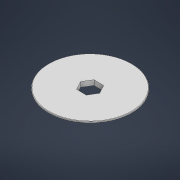
# Autodesk Inventor part: Pulley because david still hates it
Saved by Autodesk Inventor 2022 (Build 260153000, 153)
## iProperties
Created: 2022-01-21
Part Number: Pulley because david still hates it
Material: Generic
Document SubType Name: Modeling
Designer: izack
Density: 1 g/cm^3
Appearance: Default
Author: izack
## iProperties of the stored document Pulley because david hates it_3DPrint.ipt
Created: 2022-01-21
Part Number: Pulley because david hates it_3DPrint
Material: Generic
Document SubType Name: Modeling
Designer: izack
Density: 1 g/cm^3
Appearance: Default
Author: izack
Autodesk Inventor part; units mm, degrees
ref_plane "YZ Plane" through (0, 0, 0) normal (1, 0, 0) x (0, 1, 0)
ref_plane "XZ Plane" through (0, 0, 0) normal (0, 1, 0) x (-1, 0, 0)
ref_plane "XY Plane" through (0, 0, 0) normal (0, 0, 1) x (1, 0, 0)
sketch "Sketch1" plane through (0, 0, 0) normal (0, 0, 1) x (1, 0, 0)
  line L0 (0, 0) -> (12.7, 0)
  line L1 (12.7, 0) -> (12.7, 3)
  line L2 (12.7, 3) -> (0, 3)
  line L3 (0, 3) -> (0, 0)
  ellipse E0 centre (12.7, 1.5) end of major axis (9.9101, 1.5) minor radius 0.9957
  point P0 (12.7, 0.5043)
  point P1 (12.7, 2.4957)
  dimension "d0" = 12.7
  dimension "d1" = 3
  constraints: 8 end point, 3 perpendicular, 1 horizontal, 1 midpoint, 2 other
  measures "d0" distance of L0.start L0.end
  measures "d1" distance of L0.end L1.end
revolve "Revolution1" add sketch "Sketch1" angle 360 about axis through (0, 3, 0) along (0, -1, 0) contours L3 L2 L1 E0 L0
fillet "Fillet1" radius 0.127 4 edges at (-12.7, 3, 0) (-12.7, 2.4957, 0) (-12.7, 0.5043, 0) (-12.7, 0, 0)
sketch "Sketch2" plane through (0, 0, 0) normal (0, -1, 0) x (1, 0, 0)
  circle A0 centre (0, 0) radius 2.6
  line L0 (1.5658, -2.5616) -> (-1.4355, -2.6368)
  line L1 (-1.4355, -2.6368) -> (-3.0013, -0.0752)
  line L2 (-3.0013, -0.0752) -> (-1.5658, 2.5616)
  line L3 (-1.5658, 2.5616) -> (1.4355, 2.6368)
  line L4 (1.4355, 2.6368) -> (3.0013, 0.0752)
  line L5 (3.0013, 0.0752) -> (1.5658, -2.5616)
  point P0 (2.2835, -1.2432)
  dimension "d4" = 5.2
  constraints: 12 end point, 2 coincident, 1 midpoint, 16 other
extrude "Extrusion1" cut sketch "Sketch2" against normal through all
sketch "Sketch3" plane through (0, 0, 0) normal (0, -1, 0) x (1, 0, 0)
  circle A0 centre (0, 0) radius 22.3514
  constraints: 1 centre point, 1 coincident
extrude "Extrusion2" cut sketch "Sketch3" against normal blind 1.5
body "Solid1"
